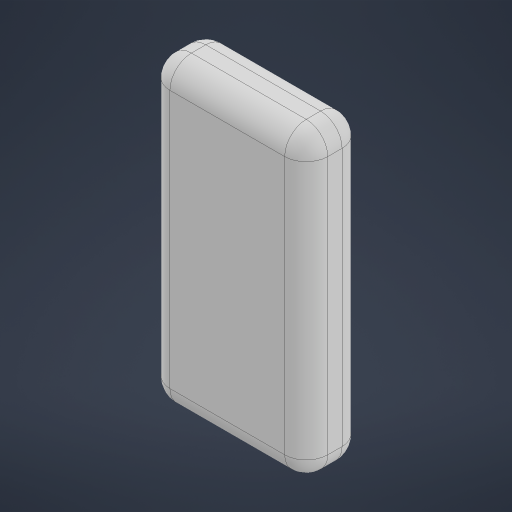
# Autodesk Inventor part: iniu_battery
Saved by Autodesk Inventor 2023 (Build 270158000, 158)
## iProperties
Created: 2024-02-26
Part Number: iniu_battery
Material: Generic
Document SubType Name: Modeling
Designer: Paul
Density: 1 g/cm^3
Appearance: Default
Author: Paul
Autodesk Inventor part; units mm, degrees
ref_plane "YZ Plane" through (0, 0, 0) normal (1, 0, 0) x (0, 1, 0)
ref_plane "XZ Plane" through (0, 0, 0) normal (0, 1, 0) x (-1, 0, 0)
ref_plane "XY Plane" through (0, 0, 0) normal (0, 0, 1) x (1, 0, 0)
sketch "Sketch1" plane through (0, 0, 0) normal (0, 0, 1) x (1, 0, 0)
  line L0 (-34.925, -66.675) -> (34.925, -66.675)
  line L1 (34.925, -66.675) -> (34.925, 66.675)
  line L2 (34.925, 66.675) -> (-34.925, 66.675)
  line L3 (-34.925, 66.675) -> (-34.925, -66.675)
  line L4 (-34.925, -66.675) -> (34.925, 66.675) construction
  line L5 (34.925, -66.675) -> (-34.925, 66.675) construction
  point P0 (0, 0)
  dimension "d0" = 69.85
  dimension "d1" = 133.35
  constraints: 12 end point, 2 midpoint, 2 parallel, 1 horizontal, 1 perpendicular
  measures "d0" distance of L1.end L2.end
  measures "d1" distance of L0.end L1.end
extrude "Extrusion1" add sketch "Sketch1" along normal blind 25.4
fillet "Fillet1" radius 9.525 12 edges at (34.925, 66.675, 12.7) (0, 66.675, 25.4) (0, 66.675, 0) (-34.925, 66.675, 12.7) (34.925, -66.675, 12.7) (34.925, 0, 25.4) (34.925, 0, 0) (-34.925, 0, 25.4) (-34.925, 0, 0) (0, -66.675, 0) (-34.925, -66.675, 12.7) (0, -66.675, 25.4)
body "Solid1"
